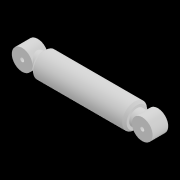
# Autodesk Inventor part: LegShock
Saved by Autodesk Inventor 2020 (Build 240168000, 168)
## iProperties
Created: 2020-05-26
Part Number: LegShock
Material: Generic
Document SubType Name: Modeling
Designer: valer
Density: 1 g/cm^3
Appearance: Default
Author: valer
Autodesk Inventor part; units mm, degrees
ref_plane "YZ Plane" through (0, 0, 0) normal (1, 0, 0) x (0, 1, 0)
ref_plane "XZ Plane" through (0, 0, 0) normal (0, 1, 0) x (-1, 0, 0)
ref_plane "XY Plane" through (0, 0, 0) normal (0, 0, 1) x (1, 0, 0)
sketch "Sketch1" plane through (0, 0, 0) normal (0, 0, 1) x (1, 0, 0)
  line L0 (0, 0) -> (229.87, 0) construction
  circle A0 centre (16.9333, 0) radius 16.9333
  circle A1 centre (212.9367, 0) radius 16.9333
  circle A2 centre (16.9333, 0) radius 3.175
  circle A3 centre (212.9367, 0) radius 3.175
  line L1 (28.1337, 12.7) -> (38.2937, 12.7)
  line L2 (38.2937, 12.7) -> (38.2937, 0)
  line L3 (38.2937, 0) -> (28.1337, 0)
  line L4 (28.1337, 0) -> (28.1337, 12.7)
  line L5 (38.2937, 12.7) -> (38.2937, 16.9333)
  line L6 (38.2937, 16.9333) -> (42.2416, 20.1303)
  line L7 (42.2416, 20.1303) -> (114.935, 20.1303)
  line L8 (114.935, 0) -> (114.935, 20.1303) construction
  line L9 (201.7363, 12.7) -> (191.5763, 12.7)
  line L10 (201.7363, 0) -> (201.7363, 12.7)
  line L11 (191.5763, 12.7) -> (191.5763, 16.9333)
  line L12 (191.5763, 16.9333) -> (187.6284, 20.1303)
  line L13 (187.6284, 20.1303) -> (114.935, 20.1303)
  line L14 (38.2937, 0) -> (201.7363, 0)
  point P0 (196.0033, 0)
  point P1 (33.8667, 0)
  dimension "d0" = 229.87
  dimension "d1" = 33.8667
  dimension "d2" = 6.35
  dimension "d3" = 6.35
  dimension "d4" = 12.7
  dimension "d5" = 10.16
  dimension "d6" = 129
  dimension "d7" = 5.08
  dimension "d8" = 4.2333
  constraints: 30 end point, 5 symmetric about line, 3 centre point, 3 perpendicular, 3 point on line, 2 coincident, 2 horizontal, 2 parallel, 2 point on circle, 2 vertical, 1 midpoint, 4 other
  measures "d0" distance of L0.start L0.end
  measures "d1" diameter of A0
  measures "d2" diameter of A2
  measures "d3" diameter of A3
  measures "d4" distance of L1.end L2.end
  measures "d5" distance of L1.start L1.end
  measures "d6" angle of L2 L6
  measures "d7" distance of L5.end L6.end
  measures "d8" distance of L1.end L5.end
revolve "Revolution1" add sketch "Sketch1" angle 360 about axis through (0, 0, 0) along (1, 0, 0) contours A0 L1 L2 L3 | L2 L5 L6 L7 L13 L12 L11 L9 A1 L14
extrude "Extrusion1" add sketch "Sketch1" along normal mid plane 25.4 contours L3 L4 A0 | A0 L4 L3 | L14 L10 A1 | A1 L10 L14
body "Solid1"
